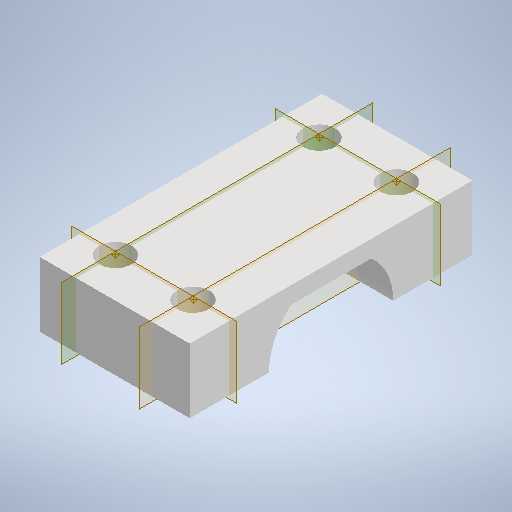
# Autodesk Inventor part: bagueSilentbloc
Saved by Autodesk Inventor 2025.2 (Build 292293000, 293)
## iProperties
Created: 2025-02-21
Part Number: bagueSilentbloc
Material: Générique
Document SubType Name: Modeling
Designer: antoi
Density: 1 g/cm^3
Appearance: Par défaut
Author: antoi
Autodesk Inventor part; units mm, degrees
ref_plane "YZ Plane" through (0, 0, 0) normal (1, 0, 0) x (0, 1, 0)
ref_plane "XZ Plane" through (0, 0, 0) normal (0, 1, 0) x (-1, 0, 0)
ref_plane "XY Plane" through (0, 0, 0) normal (0, 0, 1) x (1, 0, 0)
sketch "Esquisse1" plane through (0, 0, 0) normal (0, 1, 0) x (-1, 0, 0)
  line L0 (0, 0) -> (18.6, 0)
  line L1 (18.6, 0) -> (18.6, -35)
  line L2 (18.6, -35) -> (0, -35)
  line L3 (0, -35) -> (0, 0)
  dimension "d0" = 18.6
  dimension "d1" = 35
  constraints: 8 end point, 2 parallel, 1 horizontal, 1 perpendicular
  measures "d0" distance of L1.end L2.end
  measures "d1" distance of L0.end L1.end
extrude "Extrusion1" add sketch "Esquisse1" along normal blind 8
sketch "Esquisse2" plane through (0, 0, 0) normal (1, 0, 0) x (0, 0, -1)
  line L0 (35, 0) -> (0, 0) projected
  line L1 (25.2, 0) -> (9.8, 0)
  line L2 (22.4477, 5.9) -> (12.5523, 5.9)
  arc A0 (25.2, 0) -> (22.4477, 5.9) centre (17.5, 0) ccw
  arc A1 (12.5523, 5.9) -> (9.8, 0) centre (17.5, 0) ccw
  dimension "d5" = 5.9
  constraints: 4 end point, 4 point on circle, 2 centre point, 2 point on line, 1 midpoint, 1 parallel
  measures "d5" distance between parallel lines of L0 L2
extrude "Extrusion2" cut sketch "Esquisse2" against normal up to surface (18.6 mm away)
ref_plane "Plan de construction1" through (-18.6, 0, -4.9) normal (0, 0, 1) x (1, 0, 0)
ref_plane "Plan de construction2" through (0, 0, -30.1) normal (0, 0, -1) x (-1, 0, 0)
ref_plane "Plan de construction3" through (-14.1, 0, 0) normal (-1, 0, 0) x (0, 0, 1)
ref_plane "Plan de construction4" through (-4.5, 0, -35) normal (1, 0, 0) x (0, 0, -1)
hole "Perçage1" at (-4.5, 8, -30.1) direction (0, -1, 0) diameter 4 depth 8
hole "Perçage2" at (-14.1, 8, -30.1) direction (0, -1, 0) diameter 4 depth 8
hole "Perçage3" at (-4.5, 8, -4.9) direction (0, -1, 0) diameter 4 depth 8
hole "Perçage4" at (-14.1, 8, -4.9) direction (0, -1, 0) diameter 4 depth 8
